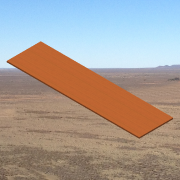
# Autodesk Inventor part: H7br
Saved by Autodesk Inventor 2014 SP1 (Build 180222100, 222)
## iProperties
Created: 2015-05-29
Part Number: H7br
Material: Wood (Cherry)
Document SubType Name: Modeling
Designer: Dave
Mass: 20069.6 g
Surface Area: 34490.3 cm^2
Volume: 31856.5 cm^3
Density: 0.63 g/cm^3
Appearance: Cherry - Natural Low Gloss
Description: 3/4" plywood @ 20" x 6.5'
Author: Dave
Autodesk Inventor part; units mm, degrees
ref_plane "YZ Plane" through (0, 0, 0) normal (1, 0, 0) x (0, 1, 0)
ref_plane "XZ Plane" through (0, 0, 0) normal (0, 1, 0) x (-1, 0, 0)
ref_plane "XY Plane" through (0, 0, 0) normal (0, 0, 1) x (1, 0, 0)
sketch "Sketch1" plane through (0, 0, 0) normal (0, 1, 0) x (-1, 0, 0)
  line L0 (0, 0) -> (1981.2, 0)
  line L1 (1981.2, 0) -> (1981.2, 508)
  line L2 (1981.2, 508) -> (0, 508)
  line L3 (0, 508) -> (0, 0)
  dimension "d0" = 1981.2
  dimension "d1" = 508
  constraints: 8 end point, 2 parallel, 1 horizontal, 1 perpendicular
  measures "d0" distance of L0.start L0.end
  measures "d1" distance of L2.end L0.start
extrude "Extrusion1" add sketch "Sketch1" along normal blind 19.05
body "Solid1"
